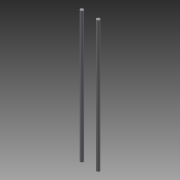
# Autodesk Inventor part: Y_Rail_Bridge-Rod-Rev1
Saved by Autodesk Inventor 2015 (Build 190159000, 159)
## iProperties
Created: 2016-12-21
Part Number: Y_Rail_Bridge-Rod-Rev1
Material: Generic
Document SubType Name: Modeling
Designer: Guy
Density: 1 g/cm^3
Appearance: Default
Author: Guy
Autodesk Inventor part; units mm, degrees
ref_plane "YZ Plane" through (0, 0, 0) normal (1, 0, 0) x (0, 1, 0)
ref_plane "XZ Plane" through (0, 0, 0) normal (0, 1, 0) x (-1, 0, 0)
ref_plane "XY Plane" through (0, 0, 0) normal (0, 0, 1) x (1, 0, 0)
sketch "Sketch1" plane through (0, 0, 0) normal (0, 0, 1) x (1, 0, 0)
  circle A0 centre (0, 0) radius 15
  circle A1 centre (150, 0) radius 15
  line L0 (0, 0) -> (150, 0)
  dimension "d0" = 30
  dimension "d3" = 30
  dimension "d4" = 150
  constraints: 2 centre point, 2 end point, 1 coincident, 1 horizontal
  measures "d0" diameter of A0
  measures "d3" diameter of A1
  measures "d4" distance of L0.end point (0, 0)
extrude "Extrusion1" add sketch "Sketch1" along normal blind 1200.8
body "Solid1"
